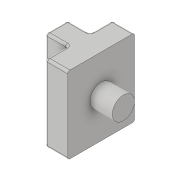
# Autodesk Inventor part: Slider2
Saved by Autodesk Inventor 2017 (Build 210142000, 142)
## iProperties
Created: 2016-07-28
Part Number: Slider2
Material: Generic
Document SubType Name: Modeling
Designer: Tutorial Books
Density: 1 g/cm^3
Appearance: Default
Author: Tutorial Books
Autodesk Inventor part; units mm, degrees
ref_plane "YZ Plane" through (0, 0, 0) normal (1, 0, 0) x (0, 1, 0)
ref_plane "XZ Plane" through (0, 0, 0) normal (0, 1, 0) x (-1, 0, 0)
ref_plane "XY Plane" through (0, 0, 0) normal (0, 0, 1) x (1, 0, 0)
sketch "Sketch1" plane through (0, 0, 0) normal (0, 1, 0) x (-1, 0, 0)
  line L0 (0, 15.24) -> (0, -15.24)
  line L1 (0, -15.24) -> (10.16, -15.24)
  line L2 (10.16, -15.24) -> (10.16, -5.08)
  line L3 (10.16, -5.08) -> (20.32, -5.08)
  line L4 (20.32, -5.08) -> (20.32, 5.08)
  line L5 (20.32, 5.08) -> (10.16, 5.08)
  line L6 (10.16, 5.08) -> (10.16, 15.24)
  line L7 (10.16, 15.24) -> (0, 15.24)
  point P0 (0, 0)
  dimension "d1" = 10.16
  dimension "d2" = 10.16
  dimension "d3" = 10.16
  dimension "d4" = 15.24
  dimension "d5" = 10.16
  constraints: 16 end point, 6 perpendicular, 2 point on line, 1 collinear, 1 midpoint, 1 vertical
  measures "d1" distance of L0.end L1.end
  measures "d2" distance of L3.end L4.end
  measures "d3" distance of L1.end L2.end
  measures "d4" distance from line of L1 point (0, 0)
  measures "d5" distance of L4.end L5.end
extrude "Extrusion1" add sketch "Sketch1" along normal blind 35.052
sketch "Sketch2" plane through (0, 0, 15.24) normal (1, 0, 0) x (0, 0, -1)
  circle A0 centre (15.24, 18.1015) radius 5.08
  point P0 (15.24, 0)
  dimension "d8" = 10.16
  constraints: 1 centre point
  measures "d8" diameter of A0
extrude "Extrusion2" add sketch "Sketch2" along normal blind 10.16
fillet "Fillet1" radius 1.016 6 edges at (-10.16, 17.526, 5.08) (-10.16, 17.526, -5.08) (-20.32, 17.526, 5.08) (-20.32, 17.526, -5.08) (-10.16, 17.526, 15.24) (-10.16, 17.526, -15.24)
fillet "Fillet2" radius 1.016 26 edges at (-9.8624, 35.052, 14.9424) (-4.572, 35.052, 15.24) (-10.4576, 35.052, 5.3776) (-15.24, 35.052, 5.08) (-20.0224, 35.052, 4.7824) (-20.32, 35.052, 0) (-20.0224, 35.052, -4.7824) (-15.24, 35.052, -5.08) (-10.4576, 35.052, -5.3776) (-10.16, 35.052, -10.16) (-9.8624, 35.052, -14.9424) (-4.572, 35.052, -15.24) (-10.16, 35.052, 10.16) (-9.8624, 0, 14.9424) (-10.16, 0, 10.16) (-10.4576, 0, 5.3776) (-15.24, 0, 5.08) (-20.0224, 0, 4.7824) (-20.32, 0, 0) (-20.0224, 0, -4.7824) (-15.24, 0, -5.08) (-10.4576, 0, -5.3776) (-10.16, 0, -10.16) (-9.8624, 0, -14.9424) (-4.572, 0, -15.24) (-4.572, 0, 15.24)
body "Solid1"
